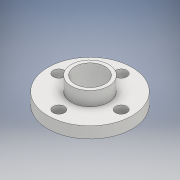
# Autodesk Inventor part: Piping_Flange_1.25in
Saved by Autodesk Inventor 2018 (Build 220112000, 112)
## iProperties
Created: 2018-10-12
Part Number: Piping_Flange_1.25in
Material: PVC-Piping
Document SubType Name: Modeling
Designer: Bradley
Density: 1.4 g/cm^3
Appearance: Smooth - White
Author: Bradley
Autodesk Inventor part; units mm, degrees
ref_plane "YZ Plane" through (0, 0, 0) normal (1, 0, 0) x (0, 1, 0)
ref_plane "XZ Plane" through (0, 0, 0) normal (0, 1, 0) x (-1, 0, 0)
ref_plane "XY Plane" through (0, 0, 0) normal (0, 0, 1) x (1, 0, 0)
sketch "Sketch1" plane through (0, 0, 0) normal (0, 1, 0) x (-1, 0, 0)
  line L0 (-16.2306, -17.907) -> (-16.2306, -13.9383)
  line L1 (-16.2306, -13.9383) -> (-21.209, -13.9383)
  line L2 (-21.209, -13.9383) -> (-21.209, 17.907)
  line L3 (-21.209, 17.907) -> (-26.162, 17.907)
  line L4 (-26.162, 17.907) -> (-26.162, -1.905)
  line L5 (-26.162, -1.905) -> (-58.7375, -1.905)
  line L6 (-58.7375, -1.905) -> (-58.7375, -17.907)
  line L7 (-58.7375, -17.907) -> (-16.2306, -17.907)
  line L8 (0, -17.907) -> (0, 17.907)
  point P0 (0, 0)
  point P1 (0, 0)
  dimension "d0" = 3.9688
  dimension "d1" = 35.814
  dimension "d2" = 42.418
  dimension "d3" = 117.475
  dimension "d4" = 52.324
  dimension "d5" = 32.4612
  dimension "d6" = 16.002
  constraints: 18 end point, 8 perpendicular, 2 point on line, 1 coincident, 1 midpoint, 1 vertical
  measures "d0" distance between parallel lines of L7 L1
  measures "d1" distance between parallel lines of L7 L3
  measures "d2" diameter of L2 L8
  measures "d3" diameter of L6 L8
  measures "d4" diameter of L4 L8
  measures "d5" diameter of L0 L8
  measures "d6" distance between parallel lines of L7 L5
revolve "Revolution1" add sketch "Sketch1" angle 360 about axis through (0, 0, -17.907) along (0, 0, 1)
sketch "Sketch2" plane through (0, 0, -1.905) normal (0, 0, 1) x (1, 0, 0)
  point P0 (0, 0)
  point P1 (0, -43.6562)
  point P2 (43.6562, 0)
  point P3 (0, 43.6562)
  point P4 (-43.6563, 0)
  dimension "d10" = 360
  dimension "d12" = 87.3125
  constraints: 1 vertical alignment, 5 other
  measures "d12" distance of point (0, 43.656) point (0, -43.656)
hole "Hole1" at (0, -43.6562, -1.905) at (43.6562, 0, -1.905) at (0, 43.6562, -1.905) at (-43.6563, 0, -1.905) direction (0, 0, -1) diameter 15.875 end through all
body "Solid1"
